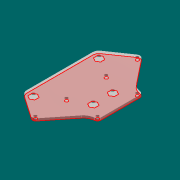
# Autodesk Inventor part: 膝_メインフレーム_6_1
Saved by Autodesk Inventor 2016 (Build 200138000, 138)
## iProperties
Created: 2016-08-23
Part Number: 膝_メインフレーム_6_1
Material: GFRP
Document SubType Name: Modeling
Designer: hiro
Density: 1.75 g/cm^3
Appearance: 滑らか - 淡い灰色
Mass: 12.3455 g
Surface Area: 77.8447 cm^2
Volume: 7.05457 cm^3
Author: hiro
Autodesk Inventor part; units mm, degrees
ref_plane "YZ Plane" through (0, 0, 0) normal (1, 0, 0) x (0, 1, 0)
ref_plane "XZ Plane" through (0, 0, 0) normal (0, 1, 0) x (-1, 0, 0)
ref_plane "XY Plane" through (0, 0, 0) normal (0, 0, 1) x (1, 0, 0)
derived "膝_基準フレーム_6_1.ipt"
sketch "スケッチ1" plane through (0, 0, 0) normal (0, 0, 1) x (1, 0, 0)
  line L0 (-16, 46.7205) -> (-16, 14.7205) construction
  line L1 (-16, 14.7205) -> (23.5, 14.7205) construction
  line L2 (-16, 46.7205) -> (23.5, 46.7205) construction
  line L3 (35.5, 41.3035) -> (35.5, 20.1375) construction
  arc A0 (35.5, 41.3035) -> (23.5, 46.7205) centre (23.5, 30.7205) ccw construction
  arc A1 (23.5, 14.7205) -> (35.5, 20.1375) centre (23.5, 30.7205) ccw construction
  circle A2 centre (23.5, 30.7205) radius 10.5 construction
  circle A3 centre (-22, 28.5) radius 1.55 construction
  circle A4 centre (10, 8.5) radius 5.05 construction
  line L4 (-22, 28.5) -> (78, 28.5) construction
  line L5 (10, 8.5) -> (110, 8.5) construction
  line L6 (10, 15.5) -> (110, 15.5) construction
  line L7 (10, 1.5) -> (110, 1.5) construction
  arc A5 (10, 15.5) -> (10, 1.5) centre (10, 8.5) ccw construction
  arc A6 (110, 1.5) -> (110, 15.5) centre (110, 8.5) ccw construction
  circle A7 centre (-22, 28.5) radius 5.5 construction
  line L8 (0, 0) -> (-46.0482, 0) construction
  arc A8 (110, -15.5) -> (110, -1.5) centre (110, -8.5) ccw construction
  line L9 (10, -1.5) -> (110, -1.5) construction
  line L10 (10, -8.5) -> (110, -8.5) construction
  line L11 (10, -15.5) -> (110, -15.5) construction
  line L12 (-22, -28.5) -> (78, -28.5) construction
  line L13 (35.5, -41.3035) -> (35.5, -20.1375) construction
  circle A9 centre (10, -8.5) radius 5.05 construction
  arc A10 (10, -1.5) -> (10, -15.5) centre (10, -8.5) ccw construction
  arc A11 (23.5, -46.7205) -> (35.5, -41.3035) centre (23.5, -30.7205) ccw construction
  arc A12 (35.5, -20.1375) -> (23.5, -14.7205) centre (23.5, -30.7205) ccw construction
  circle A13 centre (23.5, -30.7205) radius 10.5 construction
  line L14 (-16, -46.7205) -> (-16, -14.7205) construction
  line L15 (-16, -14.7205) -> (23.5, -14.7205) construction
  line L16 (-16, -46.7205) -> (23.5, -46.7205) construction
  circle A14 centre (-22, -28.5) radius 1.55 construction
  circle A15 centre (-22, -28.5) radius 5.5 construction
  line L17 (39.9042, 9.2519) -> (33.6649, 33.3521) construction
  line L18 (34.9944, 6.2689) -> (16.4805, 22.9118) construction
  arc A16 (34.9944, 6.2689) -> (39.9042, 9.2519) centre (37, 8.5) ccw construction
  arc A17 (33.6649, 33.3521) -> (16.4805, 22.9118) centre (23.5, 30.7205) ccw construction
  line L19 (37, 8.5) -> (23.5, 30.7205) construction
  line L20 (10, 8.5) -> (23.5, 30.7205) construction
  circle A18 centre (22.5, 44.2205) radius 1.35
  circle A19 centre (22.5, 17.2205) radius 1.35
  circle A20 centre (-4.5, 17.2205) radius 1.35
  line L21 (22.5, 17.2205) -> (-4.5, 17.2205) construction
  line L22 (-4.5, 17.2205) -> (-4.5, 44.2205) construction
  line L23 (-4.5, 44.2205) -> (22.5, 44.2205) construction
  line L24 (22.5, 44.2205) -> (22.5, 17.2205) construction
  circle A21 centre (23.5, 30.7205) radius 11 construction
  circle A22 centre (-22, 28.5) radius 1.55
  circle A23 centre (10, 8.5) radius 1.55
  circle A24 centre (-4.5, 44.2205) radius 1.35
  circle A25 centre (-22, -28.5) radius 1.55
  circle A26 centre (-4.5, -44.2205) radius 1.35
  circle A27 centre (-4.5, -17.2205) radius 1.35
  circle A28 centre (22.5, -17.2205) radius 1.35
  circle A29 centre (10, -8.5) radius 1.55
  circle A30 centre (22.5, -44.2205) radius 1.35
  circle A31 centre (23.5, -30.7205) radius 11 construction
  line L25 (-27.5, 28.5) -> (-27.5, -28.5)
  arc A32 (-25.1237, 33.0269) -> (-27.5, 28.5) centre (-22, 28.5) ccw
  line L26 (-25.1237, 33.0269) -> (-5.2788, 46.7205)
  line L27 (-5.2788, 46.7205) -> (-3.2946, 46.7205)
  line L28 (-3.2946, 46.7205) -> (14.8935, 23.87)
  circle A33 centre (-4.5, 44.2205) radius 2.5 construction
  arc A34 (14.8935, 23.87) -> (25, 19.8232) centre (23.5, 30.7205) ccw
  line L29 (25, 19.8232) -> (25, 14.3677)
  circle A35 centre (22.5, 17.2205) radius 2.5 construction
  line L30 (25, 14.3677) -> (25, 0.6427)
  line L31 (-25.1237, -33.0269) -> (-5.2788, -46.7205)
  arc A36 (-27.5, -28.5) -> (-25.1237, -33.0269) centre (-22, -28.5) ccw
  line L32 (-3.2946, -46.7205) -> (14.8935, -23.87)
  arc A37 (25, -19.8232) -> (14.8935, -23.87) centre (23.5, -30.7205) ccw
  line L33 (25, -19.8232) -> (25, -14.3677)
  line L34 (25, -14.3677) -> (25, 0.6427)
  line L35 (-5.2788, -46.7205) -> (-3.2946, -46.7205)
  circle A38 centre (10, 8.5) radius 5.6 construction
  circle A39 centre (-22, 28.5) radius 5.6 construction
  line L36 (23.5, 30.7205) -> (37, 52.941) construction
  circle A40 centre (23.5, 30.7205) radius 26 construction
  circle A41 centre (10, 8.5) radius 52 construction
  line L37 (23.5, 30.7205) -> (-2.4935, 30.1394) construction
  line L38 (10, 8.5) -> (-16, 53.5333) construction
  line L39 (-2.4935, 30.1394) -> (-16, 53.5333) construction
  line L40 (37, 8.5) -> (62, 8.5) construction
  point P0 (35.5, 30.7205)
  point P1 (35.5, -30.7205)
  point P2 (22.5, 30.7205)
extrude "押し出し1" add sketch "スケッチ1" along normal blind 2 contours A32 L26 L27 L28 A34 L29 L30 L34 L33 A37 L32 L35 L31 A36 L25
fillet "フィレット2" radius 3 6 edges at (-5.2788, 46.7205, 1) (-3.2946, 46.7205, 1) (25, 19.8232, 1) (25, -19.8232, 1) (-5.2788, -46.7205, 1) (-3.2946, -46.7205, 1)
sketch "スケッチ4" plane through (-27.5, -28.5, 0) normal (0, 0, -1) x (-1, 0, 0)
  circle A0 centre (-5.5, 57) radius 1.55 projected
  circle A1 centre (-37.5, 37) radius 1.55 projected
  circle A2 centre (-37.5, 20) radius 1.55 projected
  circle A3 centre (-5.5, 0) radius 1.55 projected
  line L0 (0, 57) -> (0, 0) projected
  arc A4 (0, 57) -> (-2.3763, 61.5269) centre (-5.5, 57) ccw projected
  line L1 (-2.45, 58.7609) -> (-2.45, 55.2391)
  line L2 (-2.45, 55.2391) -> (-5.5, 53.4782)
  line L3 (-5.5, 53.4782) -> (-8.55, 55.2391)
  line L4 (-8.55, 55.2391) -> (-8.55, 58.7609)
  line L5 (-8.55, 58.7609) -> (-5.5, 60.5218)
  line L6 (-5.5, 60.5218) -> (-2.45, 58.7609)
  circle A5 centre (-5.5, 59.4718) radius 1.05
  circle A6 centre (-7.6407, 58.2359) radius 1.05
  circle A7 centre (-7.6407, 55.7641) radius 1.05
  circle A8 centre (-5.5, 54.5282) radius 1.05
  circle A9 centre (-3.3593, 55.7641) radius 1.05
  circle A10 centre (-3.3593, 58.2359) radius 1.05
  line L7 (-34.45, 38.7609) -> (-34.45, 35.2391)
  line L8 (-34.45, 35.2391) -> (-37.5, 33.4782)
  line L9 (-37.5, 33.4782) -> (-40.55, 35.2391)
  line L10 (-40.55, 35.2391) -> (-40.55, 38.7609)
  line L11 (-40.55, 38.7609) -> (-37.5, 40.5218)
  line L12 (-37.5, 40.5218) -> (-34.45, 38.7609)
  circle A11 centre (-37.5, 39.4718) radius 1.05
  circle A12 centre (-39.6407, 38.2359) radius 1.05
  circle A13 centre (-39.6407, 35.7641) radius 1.05
  circle A14 centre (-37.5, 34.5282) radius 1.05
  circle A15 centre (-35.3593, 35.7641) radius 1.05
  circle A16 centre (-35.3593, 38.2359) radius 1.05
  line L13 (-39.6407, 38.2359) -> (-35.3593, 35.7641) construction
  line L14 (-39.6407, 38.2359) -> (-40.55, 38.7609) construction
  line L15 (-35.3593, 38.2359) -> (-39.6407, 35.7641) construction
  line L16 (-35.3593, 38.2359) -> (-34.45, 38.7609) construction
  line L17 (-52.5, 11.6989) -> (-52.5, 45.3011) construction
  line L18 (-52.5, 28.5) -> (0, 28.5) construction
  circle A17 centre (-5.5, 0) radius 1.55
  circle A18 centre (-37.5, 20) radius 1.55
  line L19 (-2.45, -1.7609) -> (-2.45, 1.7609)
  line L20 (-2.45, 1.7609) -> (-5.5, 3.5218)
  line L21 (-5.5, 3.5218) -> (-8.55, 1.7609)
  line L22 (-8.55, 1.7609) -> (-8.55, -1.7609)
  line L23 (-8.55, -1.7609) -> (-5.5, -3.5218)
  line L24 (-5.5, -3.5218) -> (-2.45, -1.7609)
  circle A19 centre (-5.5, -2.4718) radius 1.05
  circle A20 centre (-7.6407, -1.2359) radius 1.05
  circle A21 centre (-7.6407, 1.2359) radius 1.05
  circle A22 centre (-5.5, 2.4718) radius 1.05
  circle A23 centre (-3.3593, 1.2359) radius 1.05
  circle A24 centre (-3.3593, -1.2359) radius 1.05
  line L25 (-37.5, 23.5218) -> (-40.55, 21.7609)
  circle A25 centre (-39.6407, 21.2359) radius 1.05
  circle A26 centre (-37.5, 22.4718) radius 1.05
  circle A27 centre (-35.3593, 21.2359) radius 1.05
  line L26 (-34.45, 21.7609) -> (-37.5, 23.5218)
  line L27 (-40.55, 21.7609) -> (-40.55, 18.2391)
  circle A28 centre (-37.5, 17.5282) radius 1.05
  line L28 (-37.5, 16.4782) -> (-34.45, 18.2391)
  circle A29 centre (-35.3593, 18.7641) radius 1.05
  line L29 (-40.55, 18.2391) -> (-37.5, 16.4782)
  circle A30 centre (-39.6407, 18.7641) radius 1.05
  line L30 (-34.45, 18.2391) -> (-34.45, 21.7609)
  line L31 (-39.6407, 18.7641) -> (-35.3593, 21.2359) construction
  line L32 (-39.6407, 18.7641) -> (-40.55, 18.2391) construction
  line L33 (-35.3593, 18.7641) -> (-39.6407, 21.2359) construction
  line L34 (-35.3593, 18.7641) -> (-34.45, 18.2391) construction
  point P0 (-27.5, 28.5)
  point P1 (-8.55, 58.7609)
  point P2 (-8.55, 55.2391)
  point P3 (-5.5, 53.4782)
  point P4 (-2.45, 55.2391)
  point P5 (-2.45, 58.7609)
  point P6 (-34.45, 37)
  point P7 (-40.55, 37)
  point P8 (-8.55, -1.7609)
  point P9 (-8.55, 1.7609)
  point P10 (-5.5, 3.5218)
  point P11 (-2.45, 1.7609)
  point P12 (-2.45, -1.7609)
  point P13 (-37.5, 23.5218)
  point P14 (-34.45, 20)
  point P15 (-40.55, 20)
  dimension "d10" = 2.1
  dimension "d18" = 2.1
  dimension "d9" = 6.1
  dimension "d13" = 360
  dimension "d17" = 6.1
  constraints: 66 end point, 37 symmetric about line, 12 vertical alignment, 10 horizontal, 6 midpoint, 5 centre point, 5 equal length, 4 coincident, 2 collinear, 2 horizontal alignment, 2 point on circle, 2 vertical, 94 other
  measures "d9" distance between parallel lines of L1 L4
  measures "d17" distance between parallel lines of L7 L10
extrude "押し出し3" cut sketch "スケッチ4" against normal blind 0.5 contours A0 A10 L1 A9 | A10 A0 | A0 A10 L6 L1 | A9 L1 L2 A0 | A0 A9 | A0 A5 L6 A10 | L1 A10 | A9 L2 A8 A0 | A9 L1 | A5 A0 | A0 A5 L5 L6 | A10 L6 | A8 L2 L3 A0 | A0 A8 | L2 A9 | A0 A6 L5 A5 | L6 A5 | A8 L3 A7 A0 | A8 L2 | A6 A0 | A0 A6 L4 L5 | A5 L5 | A7 L3 L4 A0 | A0 A7 | L3 A8 | A0 A7 L4 A6 | L5 A6 | A7 L3 | A6 L4 | L4 A7 | A1 A16 L7 A15 | A16 A1 | A1 A16 L12 L7 | A15 L7 L8 A1 | A1 A15 | A1 A11 L12 A16 | L7 A16 | A15 L8 A14 A1 | A15 L7 | A11 A1 | A1 A11 L11 L12 | A16 L12 | A14 L8 L9 A1 | A1 A14 | L8 A15 | A1 A12 L11 A11 | L12 A11 | A14 L9 A13 A1 | A14 L8 | A12 A1 | A1 A12 L10 L11 | A11 L11 | A13 L9 L10 A1 | A1 A13 | L9 A14 | A1 A13 L10 A12 | L11 A12 | A13 L9 | A12 L10 | L10 A13 | A2 A27 L30 A29 | A27 A2 | A2 A27 L26 L30 | A29 L30 L28 A2 | A2 A29 | A2 A26 L26 A27 | L30 A27 | A29 L28 A28 A2 | A29 L30 | A26 A2 | A2 A26 L25 L26 | A27 L26 | A28 L28 L29 A2 | A2 A28 | L28 A29 | A2 A25 L25 A26 | L26 A26 | A28 L29 A30 A2 | A28 L28 | A25 A2 | A2 A25 L27 L25 | A26 L25 | A30 L29 L27 A2 | A2 A30 | L29 A28 | A2 A30 L27 A25 | L25 A25 | A30 L29 | A25 L27 | L27 A30 | A3 A23 L19 A24 | A23 A3 | A3 A23 L20 L19 | A24 L19 L24 A3 | A3 A24 | A3 A22 L20 A23 | L19 A23 | A24 L24 A19 A3 | A24 L19 | A22 A3 | A3 A22 L21 L20 | A23 L20 | A19 L24 L23 A3 | A3 A19 | L24 A24 | A3 A21 L21 A22 | L20 A22 | A19 L23 A20 A3 | A19 L24 | A21 A3 | A3 A21 L22 L21 | A22 L21 | A20 L23 L22 A3 | A3 A20 | L23 A19 | A3 A20 L22 A21 | L21 A21 | A20 L23 | A21 L22 | L22 A20
equation "\"d9\" = d17"
